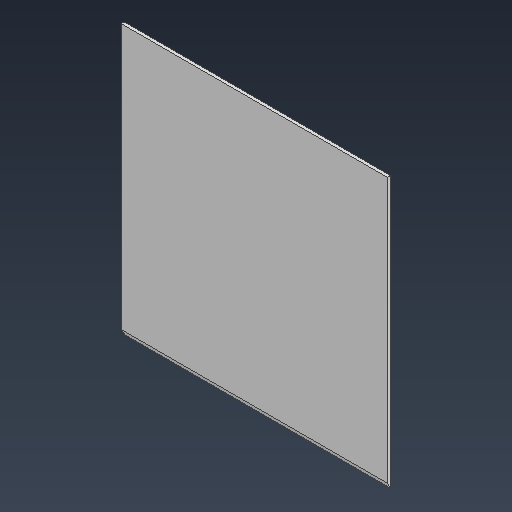
# Autodesk Inventor part: наклон
Saved by Autodesk Inventor 2025.2 (Build 292293000, 293)
## iProperties
Created: 2025-09-06
Part Number: наклон
Material: Типовые
Document SubType Name: Modeling
Designer: Trene
Density: 1 g/cm^3
Appearance: По умолчанию
Author: Trene
Autodesk Inventor part; units mm, degrees
ref_plane "YZ Plane" through (0, 0, 0) normal (1, 0, 0) x (0, 1, 0)
ref_plane "XZ Plane" through (0, 0, 0) normal (0, 1, 0) x (-1, 0, 0)
ref_plane "XY Plane" through (0, 0, 0) normal (0, 0, 1) x (1, 0, 0)
sketch "Эскиз1" plane through (0, 0, 0) normal (0, 0, 1) x (1, 0, 0)
  line L0 (0, 0) -> (130, 0)
  line L1 (130, 0) -> (130, 140)
  line L2 (130, 140) -> (0, 140)
  line L3 (0, 140) -> (0, 0)
  dimension "d0" = 130
  dimension "d1" = 140
  constraints: 8 end point, 2 parallel, 1 horizontal, 1 perpendicular
  measures "d0" distance of L2.end L1.end
  measures "d1" distance of L1.end L0.end
extrude "Выдавливание1" add sketch "Эскиз1" along normal blind 1.5
sketch "Эскиз2" plane through (0, 0, 0) normal (-1, 0, 0) x (0, 0, 1)
  line L0 (1.5, 0) -> (1.5, 140) projected
  line L1 (-41.9118, 21.1155) -> (-83.4972, 43.0167) projected
  line L2 (1.5, 0) -> (-2.924, 2.3299)
  line L3 (-2.924, 2.3299) -> (11.3571, 29.4464)
  line L4 (150.8042, 338.7544) -> (-21.6092, 11.3806) projected
  line L5 (-2.924, 2.3299) -> (0.6125, -7.5611)
  line L6 (0.6125, -7.5611) -> (16.5418, 17.4148)
  line L7 (16.5418, 17.4148) -> (9.9779, 26.8277)
  point P0 (0, 0)
  dimension "d4" = 5
  constraints: 10 end point, 2 parallel, 1 point on line
  measures "d4" distance of L0.start L2.end
extrude "Выдавливание2" cut sketch "Эскиз2" against normal through all
